Autodesk Fusion 360 part; units mm, degrees
note: some values were not read from the file. Chosen so that the rebuilt part matches the saved one: which face or edge a step refers to; which pieces of a blend or face edit are solid. Set by a fixed rule: which sketch regions a step uses.
(part 2 of 2)
sketch "Sketch14" plane through (0, 6.1, 0) normal (0, 1, 0) x (-1, 0, 0)
  line L0 (1, 7.8) -> (-21.04, 7.8)
  line L1 (-20.84, 4.25) -> (0.8, 4.25) construction
  line L2 (-10.02, 7.8) -> (-10.02, 0.2) construction
  spline S0 degree 3 poles (-10.1584, 7.1337) (-10.2189, 7.0606) (-10.2819, 6.9799) (-10.302, 6.9572) knots 0 0 0 0 1 1 1 1
  spline S1 degree 3 poles (-10.302, 6.9572) (-10.3373, 6.9144) (-10.3222, 6.9119) (-10.0172, 6.9119) knots 0 0 0 0 1 1 1 1
  line L3 (-10.0172, 6.9119) -> (-9.697, 6.9119)
  line L4 (-9.697, 6.9119) -> (-9.818, 7.0581)
  spline S2 degree 3 poles (-9.818, 7.0581) (-9.9441, 7.2068) (-10.0021, 7.2648) (-10.0323, 7.2648) knots 0 0 0 0 1 1 1 1
  spline S3 degree 3 poles (-10.0323, 7.2648) (-10.0424, 7.2648) (-10.0979, 7.2043) (-10.1584, 7.1337) knots 0 0 0 0 1 1 1 1
  spline S4 degree 3 poles (-11.6481, 6.2766) (-12.0111, 5.8405) (-12.0968, 5.7347) (-12.0968, 5.7246) knots 0 0 0 0 1 1 1 1
  spline S5 degree 3 poles (-12.0968, 5.7246) (-12.0968, 5.7195) (-11.9254, 5.7195) (-11.7162, 5.7271) knots 0 0 0 0 1 1 1 1
  line L5 (-11.7162, 5.7271) -> (-11.3381, 5.7397)
  line L6 (-11.3381, 5.7397) -> (-11.3381, 6.0372)
  spline S6 degree 3 poles (-11.3381, 6.0372) (-11.3381, 6.1985) (-11.3381, 6.3825) (-11.3406, 6.4455) knots 0 0 0 0 1 1 1 1
  spline S7 degree 3 poles (-11.3406, 6.4455) (-11.3406, 6.5262) (-11.3507, 6.559) (-11.3759, 6.559) knots 0 0 0 0 1 1 1 1
  spline S8 degree 3 poles (-11.3759, 6.559) (-11.3961, 6.559) (-11.5196, 6.4304) (-11.6481, 6.2766) knots 0 0 0 0 1 1 1 1
  spline S9 degree 3 poles (-10.2567, 6.327) (-10.36, 6.201) (-10.5188, 6.017) (-10.6096, 5.9187) knots 0 0 0 0 1 1 1 1
  line L7 (-10.6096, 5.9187) -> (-10.7734, 5.7397)
  line L8 (-10.7734, 5.7397) -> (-10.3877, 5.7321)
  spline S10 degree 3 poles (-10.3877, 5.7321) (-10.176, 5.7296) (-9.8357, 5.7296) (-9.6315, 5.7321) knots 0 0 0 0 1 1 1 1
  line L9 (-9.6315, 5.7321) -> (-9.261, 5.7397)
  line L10 (-9.261, 5.7397) -> (-9.4248, 5.9187)
  spline S11 degree 3 poles (-9.4248, 5.9187) (-9.5156, 6.0145) (-9.6769, 6.201) (-9.7853, 6.327) knots 0 0 0 0 1 1 1 1
  spline S12 degree 3 poles (-9.7853, 6.327) (-9.8937, 6.4556) (-9.9995, 6.559) (-10.0248, 6.559) knots 0 0 0 0 1 1 1 1
  spline S13 degree 3 poles (-10.0248, 6.559) (-10.0474, 6.559) (-10.1533, 6.4556) (-10.2567, 6.327) knots 0 0 0 0 1 1 1 1
  spline S14 degree 3 poles (-8.6963, 6.2943) (-8.6963, 6.1481) (-8.6988, 5.9641) (-8.6988, 5.8859) knots 0 0 0 0 1 1 1 1
  line L11 (-8.6988, 5.8859) -> (-8.7013, 5.7397)
  line L12 (-8.7013, 5.7397) -> (-8.3182, 5.7271)
  spline S15 degree 3 poles (-8.3182, 5.7271) (-8.109, 5.7195) (-7.9375, 5.7195) (-7.9375, 5.7271) knots 0 0 0 0 1 1 1 1
  spline S16 degree 3 poles (-7.9375, 5.7271) (-7.9401, 5.7649) (-8.6257, 6.559) (-8.656, 6.559) knots 0 0 0 0 1 1 1 1
  spline S17 degree 3 poles (-8.656, 6.559) (-8.6862, 6.559) (-8.6938, 6.5111) (-8.6963, 6.2943) knots 0 0 0 0 1 1 1 1
  spline S18 degree 3 poles (-11.5171, 5.1927) (-11.5902, 5.1045) (-11.6683, 5.0162) (-11.691, 4.9961) knots 0 0 0 0 1 1 1 1
  spline S19 degree 3 poles (-11.691, 4.9961) (-11.7137, 4.9759) (-11.8246, 4.8473) (-11.938, 4.7112) knots 0 0 0 0 1 1 1 1
  spline S20 degree 3 poles (-11.938, 4.7112) (-12.1624, 4.444) (-12.2128, 4.3306) (-12.1876, 4.144) knots 0 0 0 0 1 1 1 1
  spline S21 degree 3 poles (-12.1876, 4.144) (-12.1674, 4.0029) (-12.1397, 3.955) (-12.0288, 3.8693) knots 0 0 0 0 1 1 1 1
  spline S22 degree 3 poles (-12.0288, 3.8693) (-11.9481, 3.8063) (-11.9153, 3.7987) (-11.7591, 3.7987) knots 0 0 0 0 1 1 1 1
  spline S23 degree 3 poles (-11.7591, 3.7987) (-11.6607, 3.7987) (-11.5498, 3.8063) (-11.5095, 3.8189) knots 0 0 0 0 1 1 1 1
  spline S24 degree 3 poles (-11.5095, 3.8189) (-11.4213, 3.8441) (-11.4187, 3.8012) (-11.5045, 3.6348) knots 0 0 0 0 1 1 1 1
  line L13 (-11.5045, 3.6348) -> (-11.5675, 3.5088)
  line L14 (-11.5675, 3.5088) -> (-11.4792, 3.5063)
  spline S25 degree 3 poles (-11.4792, 3.5063) (-11.4314, 3.5038) (-11.3784, 3.5012) (-11.3658, 3.4987) knots 0 0 0 0 1 1 1 1
  spline S26 degree 3 poles (-11.3658, 3.4987) (-11.3482, 3.4962) (-11.3381, 3.8088) (-11.333, 4.4239) knots 0 0 0 0 1 1 1 1
  spline S27 degree 3 poles (-11.333, 4.4239) (-11.3305, 5.0818) (-11.3356, 5.349) (-11.3557, 5.349) knots 0 0 0 0 1 1 1 1
  spline S28 degree 3 poles (-11.3557, 5.349) (-11.3709, 5.349) (-11.444, 5.2784) (-11.5171, 5.1927) knots 0 0 0 0 1 1 1 1
  spline S29 degree 3 poles (-10.413, 4.9557) (-10.597, 4.739) (-10.781, 4.5096) (-10.8188, 4.4465) knots 0 0 0 0 1 1 1 1
  spline S30 degree 3 poles (-10.8188, 4.4465) (-10.96, 4.2247) (-10.8919, 3.9903) (-10.6474, 3.8466) knots 0 0 0 0 1 1 1 1
  spline S31 degree 3 poles (-10.6474, 3.8466) (-10.544, 3.7861) (-10.5138, 3.7811) (-10.3751, 3.7937) knots 0 0 0 0 1 1 1 1
  spline S32 degree 3 poles (-10.3751, 3.7937) (-10.2894, 3.8012) (-10.1911, 3.8163) (-10.1584, 3.8264) knots 0 0 0 0 1 1 1 1
  spline S33 degree 3 poles (-10.1584, 3.8264) (-10.1029, 3.8441) (-10.1004, 3.839) (-10.1155, 3.7735) knots 0 0 0 0 1 1 1 1
  spline S34 degree 3 poles (-10.1155, 3.7735) (-10.1306, 3.713) (-10.1936, 3.5567) (-10.2239, 3.5088) knots 0 0 0 0 1 1 1 1
  spline S35 degree 3 poles (-10.2239, 3.5088) (-10.2289, 3.5012) (-10.1357, 3.4962) (-10.0172, 3.4962) knots 0 0 0 0 1 1 1 1
  spline S36 degree 3 poles (-10.0172, 3.4962) (-9.8987, 3.4962) (-9.8054, 3.5012) (-9.8105, 3.5088) knots 0 0 0 0 1 1 1 1
  spline S37 degree 3 poles (-9.8105, 3.5088) (-9.8483, 3.5743) (-9.929, 3.7735) (-9.929, 3.8037) knots 0 0 0 0 1 1 1 1
  spline S38 degree 3 poles (-9.929, 3.8037) (-9.929, 3.8315) (-9.9138, 3.839) (-9.871, 3.8264) knots 0 0 0 0 1 1 1 1
  spline S39 degree 3 poles (-9.871, 3.8264) (-9.8407, 3.8163) (-9.7424, 3.8012) (-9.6517, 3.7937) knots 0 0 0 0 1 1 1 1
  spline S40 degree 3 poles (-9.6517, 3.7937) (-9.4979, 3.7811) (-9.4803, 3.7861) (-9.3643, 3.8642) knots 0 0 0 0 1 1 1 1
  spline S41 degree 3 poles (-9.3643, 3.8642) (-9.2156, 3.9676) (-9.1475, 4.0861) (-9.1475, 4.2398) knots 0 0 0 0 1 1 1 1
  spline S42 degree 3 poles (-9.1475, 4.2398) (-9.1475, 4.3835) (-9.1904, 4.4491) (-9.6214, 4.9557) knots 0 0 0 0 1 1 1 1
  spline S43 degree 3 poles (-9.6214, 4.9557) (-9.8811, 5.2608) (-9.9693, 5.349) (-10.0172, 5.349) knots 0 0 0 0 1 1 1 1
  spline S44 degree 3 poles (-10.0172, 5.349) (-10.0651, 5.349) (-10.1533, 5.2608) (-10.413, 4.9557) knots 0 0 0 0 1 1 1 1
  line L15 (-8.7064, 4.4289) -> (-8.7064, 3.5088)
  line L16 (-8.7064, 3.5088) -> (-8.5829, 3.5088)
  line L17 (-8.5829, 3.5088) -> (-8.4619, 3.5088)
  line L18 (-8.4619, 3.5088) -> (-8.5047, 3.5743)
  spline S45 degree 3 poles (-8.5047, 3.5743) (-8.5274, 3.6096) (-8.5627, 3.6853) (-8.5829, 3.7407) knots 0 0 0 0 1 1 1 1
  spline S46 degree 3 poles (-8.5829, 3.7407) (-8.6182, 3.8415) (-8.6182, 3.8415) (-8.5602, 3.8239) knots 0 0 0 0 1 1 1 1
  spline S47 degree 3 poles (-8.5602, 3.8239) (-8.5299, 3.8163) (-8.424, 3.8012) (-8.3283, 3.7962) knots 0 0 0 0 1 1 1 1
  spline S48 degree 3 poles (-8.3283, 3.7962) (-8.177, 3.7861) (-8.1392, 3.7911) (-8.0535, 3.8415) knots 0 0 0 0 1 1 1 1
  spline S49 degree 3 poles (-8.0535, 3.8415) (-7.8922, 3.9373) (-7.8493, 4.0155) (-7.8518, 4.2096) knots 0 0 0 0 1 1 1 1
  spline S50 degree 3 poles (-7.8518, 4.2096) (-7.8518, 4.3029) (-7.8644, 4.4037) (-7.8821, 4.4314) knots 0 0 0 0 1 1 1 1
  spline S51 degree 3 poles (-7.8821, 4.4314) (-7.9451, 4.5474) (-8.6434, 5.349) (-8.6812, 5.349) knots 0 0 0 0 1 1 1 1
  spline S52 degree 3 poles (-8.6812, 5.349) (-8.6988, 5.349) (-8.7064, 5.0339) (-8.7064, 4.4289) knots 0 0 0 0 1 1 1 1
  spline S53 degree 3 poles (-12.6917, 4.56) (-12.8077, 4.4289) (-12.8682, 4.26) (-12.8405, 4.144) knots 0 0 0 0 1 1 1 1
  spline S54 degree 3 poles (-12.8405, 4.144) (-12.8329, 4.1012) (-12.7724, 4.013) (-12.7069, 3.9449) knots 0 0 0 0 1 1 1 1
  line L19 (-12.7069, 3.9449) -> (-12.5884, 3.8239)
  line L20 (-12.5884, 3.8239) -> (-12.5808, 4.0457)
  spline S55 degree 3 poles (-12.5808, 4.0457) (-12.5783, 4.1667) (-12.5783, 4.3608) (-12.5808, 4.4717) knots 0 0 0 0 1 1 1 1
  line L21 (-12.5808, 4.4717) -> (-12.5884, 4.6785)
  line L22 (-12.5884, 4.6785) -> (-12.6917, 4.56)
  line L23 (-7.4586, 4.255) -> (-7.4586, 3.834)
  line L24 (-7.4586, 3.834) -> (-7.3855, 3.8844)
  spline S56 degree 3 poles (-7.3855, 3.8844) (-7.1435, 4.0583) (-7.141, 4.376) (-7.3804, 4.6028) knots 0 0 0 0 1 1 1 1
  line L25 (-7.3804, 4.6028) -> (-7.4586, 4.6785)
  line L26 (-7.4586, 4.6785) -> (-7.4586, 4.255)
  spline S57 degree 3 poles (-10.8692, 3.1382) (-10.8793, 3.1307) (-10.8869, 3.0677) (-10.8869, 2.9996) knots 0 0 0 0 1 1 1 1
  spline S58 degree 3 poles (-10.8869, 2.9996) (-10.8869, 2.8559) (-10.8138, 2.7374) (-10.6676, 2.6492) knots 0 0 0 0 1 1 1 1
  spline S59 degree 3 poles (-10.6676, 2.6492) (-10.5869, 2.5988) (-10.5566, 2.5963) (-10.3399, 2.6089) knots 0 0 0 0 1 1 1 1
  spline S60 degree 3 poles (-10.3399, 2.6089) (-10.0701, 2.6265) (-10.0777, 2.6366) (-10.1836, 2.4148) knots 0 0 0 0 1 1 1 1
  spline S61 degree 3 poles (-10.1836, 2.4148) (-10.2113, 2.3593) (-10.2315, 2.3114) (-10.2315, 2.3064) knots 0 0 0 0 1 1 1 1
  spline S62 degree 3 poles (-10.2315, 2.3064) (-10.2315, 2.3013) (-10.1357, 2.2988) (-10.0197, 2.2988) knots 0 0 0 0 1 1 1 1
  line L27 (-10.0197, 2.2988) -> (-9.8054, 2.2988)
  line L28 (-9.8054, 2.2988) -> (-9.8685, 2.4375)
  spline S63 degree 3 poles (-9.8685, 2.4375) (-9.9012, 2.5156) (-9.929, 2.5887) (-9.929, 2.6013) knots 0 0 0 0 1 1 1 1
  spline S64 degree 3 poles (-9.929, 2.6013) (-9.929, 2.6164) (-9.8332, 2.619) (-9.6895, 2.6089) knots 0 0 0 0 1 1 1 1
  spline S65 degree 3 poles (-9.6895, 2.6089) (-9.4626, 2.5938) (-9.4475, 2.5963) (-9.3517, 2.6593) knots 0 0 0 0 1 1 1 1
  spline S66 degree 3 poles (-9.3517, 2.6593) (-9.2105, 2.7551) (-9.1425, 2.8736) (-9.1526, 3.0223) knots 0 0 0 0 1 1 1 1
  line L29 (-9.1526, 3.0223) -> (-9.1601, 3.1433)
  line L30 (-9.1601, 3.1433) -> (-10.0071, 3.1509)
  spline S67 degree 3 poles (-10.0071, 3.1509) (-10.4709, 3.1534) (-10.8591, 3.1483) (-10.8692, 3.1382) knots 0 0 0 0 1 1 1 1
  spline S68 degree 3 poles (-8.6761, 3.1382) (-8.6862, 3.1307) (-8.6938, 2.9366) (-8.6938, 2.7097) knots 0 0 0 0 1 1 1 1
  line L31 (-8.6938, 2.7097) -> (-8.6938, 2.2988)
  line L32 (-8.6938, 2.2988) -> (-8.5703, 2.2988)
  line L33 (-8.5703, 2.2988) -> (-8.4442, 2.2988)
  line L34 (-8.4442, 2.2988) -> (-8.5198, 2.44)
  spline S69 degree 3 poles (-8.5198, 2.44) (-8.6257, 2.6417) (-8.6232, 2.6442) (-8.4215, 2.6164) knots 0 0 0 0 1 1 1 1
  spline S70 degree 3 poles (-8.4215, 2.6164) (-8.1871, 2.5837) (-8.0787, 2.6089) (-7.9552, 2.7248) knots 0 0 0 0 1 1 1 1
  spline S71 degree 3 poles (-7.9552, 2.7248) (-7.8569, 2.8156) (-7.8518, 2.8307) (-7.8417, 2.9895) knots 0 0 0 0 1 1 1 1
  line L35 (-7.8417, 2.9895) -> (-7.8317, 3.1559)
  line L36 (-7.8317, 3.1559) -> (-8.2451, 3.1559)
  spline S72 degree 3 poles (-8.2451, 3.1559) (-8.4745, 3.1559) (-8.6686, 3.1483) (-8.6761, 3.1382) knots 0 0 0 0 1 1 1 1
  spline S73 degree 3 poles (-12.1977, 3.0097) (-12.1977, 2.8736) (-12.1347, 2.7576) (-12.0137, 2.6669) knots 0 0 0 0 1 1 1 1
  spline S74 degree 3 poles (-12.0137, 2.6669) (-11.9506, 2.6215) (-11.9078, 2.6139) (-11.696, 2.6164) knots 0 0 0 0 1 1 1 1
  line L37 (-11.696, 2.6164) -> (-11.449, 2.619)
  line L38 (-11.449, 2.619) -> (-11.4515, 2.5534)
  spline S75 degree 3 poles (-11.4515, 2.5534) (-11.4515, 2.5181) (-11.4616, 2.4828) (-11.4692, 2.4753) knots 0 0 0 0 1 1 1 1
  spline S76 degree 3 poles (-11.4692, 2.4753) (-11.4792, 2.4677) (-11.5095, 2.4223) (-11.5372, 2.3719) knots 0 0 0 0 1 1 1 1
  line L39 (-11.5372, 2.3719) -> (-11.5876, 2.2812)
  line L40 (-11.5876, 2.2812) -> (-11.4717, 2.2938)
  spline S77 degree 3 poles (-11.4717, 2.2938) (-11.4061, 2.2988) (-11.3507, 2.3064) (-11.3482, 2.3089) knots 0 0 0 0 1 1 1 1
  spline S78 degree 3 poles (-11.3482, 2.3089) (-11.3456, 2.3114) (-11.3406, 2.4954) (-11.3381, 2.7148) knots 0 0 0 0 1 1 1 1
  line L41 (-11.3381, 2.7148) -> (-11.3356, 3.1181)
  line L42 (-11.3356, 3.1181) -> (-11.7666, 3.1256)
  line L43 (-11.7666, 3.1256) -> (-12.1977, 3.1307)
  line L44 (-12.1977, 3.1307) -> (-12.1977, 3.0097)
  spline S79 degree 3 poles (-10.1054, 1.9257) (-10.1054, 1.9005) (-10.1382, 1.8174) (-10.181, 1.7367) knots 0 0 0 0 1 1 1 1
  line L45 (-10.181, 1.7367) -> (-10.2541, 1.593)
  line L46 (-10.2541, 1.593) -> (-10.0298, 1.593)
  spline S80 degree 3 poles (-10.0298, 1.593) (-9.9038, 1.593) (-9.8029, 1.598) (-9.8029, 1.6031) knots 0 0 0 0 1 1 1 1
  spline S81 degree 3 poles (-9.8029, 1.6031) (-9.8029, 1.6081) (-9.8307, 1.6737) (-9.8659, 1.7493) knots 0 0 0 0 1 1 1 1
  spline S82 degree 3 poles (-9.8659, 1.7493) (-9.9012, 1.8224) (-9.929, 1.9031) (-9.929, 1.9283) knots 0 0 0 0 1 1 1 1
  spline S83 degree 3 poles (-9.929, 1.9283) (-9.929, 1.961) (-9.9491, 1.9711) (-10.0172, 1.9711) knots 0 0 0 0 1 1 1 1
  spline S84 degree 3 poles (-10.0172, 1.9711) (-10.0853, 1.9711) (-10.1054, 1.961) (-10.1054, 1.9257) knots 0 0 0 0 1 1 1 1
  line L47 (-21.04, 7.8) -> (-21.04, 0)
  line L48 (-21.04, 0) -> (1, 0)
  line L49 (1, 0) -> (1, 7.8)
  constraint midpoint L0 L2.start
extrude "Extrude23" add sketch "Sketch14" along normal blind 0.3 contours S0 S1 L3 L4 S2 S3 | S4 S5 L5 L6 S6 S7 S8 | S9 L7 L8 S10 L9 L10 S11 S12 S13 | S14 L11 L12 S15 S16 S17 | S18 S19 S20 S21 S22 S23 S24 L13 L14 S25 S26 S27 S28 | S29 S30 S31 S32 S33 S34 S35 S36 S37 S38 S39 S40 S41 S42 S43 S44 | L15 L16 L17 L18 S45 S46 S47 S48 S49 S50 S51 S52 | S53 S54 L19 L20 S55 L21 L22 | L23 L24 S56 L25 L26 | S57 S58 S59 S60 S61 S62 L27 L28 S63 S64 S65 S66 L29 L30 S67 | S68 L31 L32 L33 L34 S69 S70 S71 L35 L36 S72 | S73 S74 L37 L38 S75 S76 L39 L40 S77 S78 L41 L42 L43 L44 | S79 L45 L46 S80 S81 S82 S83 S84
extrude "Extrude24" cut 1 faces at (-0.8348, -0.8228, 0.2) along direction (0, 0, -1) blind 3
sketch "Sketch15" plane through (21.04, 0, 0) normal (1, 0, 0) x (0, 1, 0)
  line L0 (6.1, 7.8) -> (-1, 7.8)
  line L1 (2.4054, 2.652) -> (3.5519, 5.6541)
  line L2 (3.5519, 5.6541) -> (3.9796, 5.6549)
  line L3 (3.9796, 5.6549) -> (5.2131, 2.6572)
  line L4 (5.2131, 2.6572) -> (4.7608, 2.6564)
  line L5 (4.7608, 2.6564) -> (4.4092, 3.5643)
  line L6 (4.4092, 3.5643) -> (3.1547, 3.562)
  line L7 (3.1547, 3.562) -> (2.827, 2.6528)
  line L8 (2.827, 2.6528) -> (2.4054, 2.652)
  line L9 (-0.1973, 3.611) -> (0.1771, 3.6444)
  spline S0 degree 3 poles (0.1771, 3.6444) (0.1878, 3.5746) (0.2078, 3.444) (0.2711, 3.3282) (0.3006, 3.2742) knots 0 0 0 0 0.020982 0.039288 0.039288 0.039288 0.039288
  spline S1 degree 3 poles (0.3006, 3.2742) (0.3399, 3.2279) (0.424, 3.1287) (0.5413, 3.0718) (0.6039, 3.0415) knots 0 0 0 0 0.018019 0.038604 0.038604 0.038604 0.038604
  spline S2 degree 3 poles (0.6039, 3.0415) (0.6757, 3.016) (0.8246, 2.9631) (0.9826, 2.9573) (1.0645, 2.9544) knots 0 0 0 0 0.022722 0.047123 0.047123 0.047123 0.047123
  spline S3 degree 3 poles (1.0645, 2.9544) (1.1363, 2.9567) (1.2732, 2.9612) (1.4035, 3.0029) (1.4654, 3.0227) knots 0 0 0 0 0.021451 0.040849 0.040849 0.040849 0.040849
  spline S4 degree 3 poles (1.4654, 3.0227) (1.5185, 3.0458) (1.6177, 3.0891) (1.6895, 3.1698) (1.7229, 3.2073) knots 0 0 0 0 0.017118 0.032023 0.032023 0.032023 0.032023
  spline S5 degree 3 poles (1.7229, 3.2073) (1.7479, 3.2474) (1.7972, 3.3266) (1.8047, 3.4195) (1.8084, 3.4653) knots 0 0 0 0 0.013958 0.027533 0.027533 0.027533 0.027533
  spline S6 degree 3 poles (1.8084, 3.4653) (1.8051, 3.5105) (1.7987, 3.5995) (1.75, 3.6741) (1.7261, 3.7107) knots 0 0 0 0 0.013357 0.026267 0.026267 0.026267 0.026267
  spline S7 degree 3 poles (1.7261, 3.7107) (1.6915, 3.7457) (1.6142, 3.8238) (1.5121, 3.8653) (1.4556, 3.8883) knots 0 0 0 0 0.014598 0.03265 0.03265 0.03265 0.03265
  spline S8 degree 3 poles (1.4556, 3.8883) (1.3911, 3.9087) (1.2152, 3.9646) (1.0352, 4.0062) (0.9212, 4.0326) knots 0 0 0 0 0.020292 0.05537 0.05537 0.05537 0.05537
  spline S9 degree 3 poles (0.9212, 4.0326) (0.8028, 4.0609) (0.6046, 4.1084) (0.4171, 4.1878) (0.3418, 4.2197) knots 0 0 0 0 0.036466 0.060986 0.060986 0.060986 0.060986
  spline S10 degree 3 poles (0.3418, 4.2197) (0.2757, 4.2577) (0.1504, 4.3297) (0.0618, 4.4436) (0.02, 4.4974) knots 0 0 0 0 0.022603 0.04287 0.04287 0.04287 0.04287
  spline S11 degree 3 poles (0.02, 4.4974) (-0.0106, 4.5553) (-0.0724, 4.6725) (-0.0808, 4.8048) (-0.0851, 4.8717) knots 0 0 0 0 0.019401 0.03927 0.03927 0.03927 0.03927
  spline S12 degree 3 poles (-0.0851, 4.8717) (-0.0797, 4.9465) (-0.0687, 5.0973) (0.0056, 5.2291) (0.043, 5.2956) knots 0 0 0 0 0.022183 0.04477 0.04477 0.04477 0.04477
  spline S13 degree 3 poles (0.043, 5.2956) (0.0921, 5.3584) (0.1937, 5.4882) (0.3423, 5.56) (0.419, 5.5971) knots 0 0 0 0 0.023577 0.048769 0.048769 0.048769 0.048769
  spline S14 degree 3 poles (0.419, 5.5971) (0.5053, 5.6271) (0.6835, 5.689) (0.872, 5.6966) (0.9693, 5.7005) knots 0 0 0 0 0.027246 0.056264 0.056264 0.056264 0.056264
  spline S15 degree 3 poles (0.9693, 5.7005) (1.0749, 5.6971) (1.2762, 5.6906) (1.4664, 5.6245) (1.5568, 5.5931) knots 0 0 0 0 0.031478 0.060031 0.060031 0.060031 0.060031
  spline S16 degree 3 poles (1.5568, 5.5931) (1.6365, 5.5545) (1.7917, 5.4795) (1.8984, 5.3444) (1.9503, 5.2787) knots 0 0 0 0 0.026183 0.050954 0.050954 0.050954 0.050954
  spline S17 degree 3 poles (1.9503, 5.2787) (1.9909, 5.2062) (2.0732, 5.0592) (2.09, 4.8914) (2.0985, 4.8062) knots 0 0 0 0 0.024624 0.04999 0.04999 0.04999 0.04999
  line L10 (2.0985, 4.8062) -> (1.7179, 4.7769)
  spline S18 degree 3 poles (1.7179, 4.7769) (1.7034, 4.8642) (1.676, 5.0286) (1.562, 5.1495) (1.5084, 5.2062) knots 0 0 0 0 0.025863 0.048747 0.048747 0.048747 0.048747
  spline S19 degree 3 poles (1.5084, 5.2062) (1.4373, 5.2483) (1.2771, 5.3432) (1.0902, 5.3479) (0.9863, 5.3506) knots 0 0 0 0 0.024412 0.054967 0.054967 0.054967 0.054967
  spline S20 degree 3 poles (0.9863, 5.3506) (0.8799, 5.3487) (0.6931, 5.3454) (0.5305, 5.2553) (0.4606, 5.2166) knots 0 0 0 0 0.031333 0.054977 0.054977 0.054977 0.054977
  spline S21 degree 3 poles (0.4606, 5.2166) (0.413, 5.1716) (0.3209, 5.0848) (0.3051, 4.9595) (0.2975, 4.8991) knots 0 0 0 0 0.018984 0.036703 0.036703 0.036703 0.036703
  spline S22 degree 3 poles (0.2975, 4.8991) (0.3023, 4.8477) (0.3118, 4.746) (0.3806, 4.6706) (0.4147, 4.6332) knots 0 0 0 0 0.01502 0.029764 0.029764 0.029764 0.029764
  spline S23 degree 3 poles (0.4147, 4.6332) (0.4826, 4.5954) (0.6692, 4.4916) (0.8791, 4.4475) (1.0126, 4.4195) knots 0 0 0 0 0.023224 0.0638 0.0638 0.0638 0.0638
  spline S24 degree 3 poles (1.0126, 4.4195) (1.15, 4.3894) (1.3758, 4.34) (1.593, 4.2613) (1.678, 4.2304) knots 0 0 0 0 0.042125 0.069241 0.069241 0.069241 0.069241
  spline S25 degree 3 poles (1.678, 4.2304) (1.7581, 4.1899) (1.9082, 4.114) (2.0154, 3.9846) (2.0654, 3.9242) knots 0 0 0 0 0.026576 0.049849 0.049849 0.049849 0.049849
  spline S26 degree 3 poles (2.0654, 3.9242) (2.1019, 3.8596) (2.1766, 3.7276) (2.1861, 3.5762) (2.191, 3.4988) knots 0 0 0 0 0.021947 0.044875 0.044875 0.044875 0.044875
  spline S27 degree 3 poles (2.191, 3.4988) (2.1851, 3.4196) (2.1731, 3.2587) (2.0946, 3.1178) (2.0547, 3.0463) knots 0 0 0 0 0.023529 0.047766 0.047766 0.047766 0.047766
  spline S28 degree 3 poles (2.0547, 3.0463) (2.0028, 2.9792) (1.8956, 2.8405) (1.7405, 2.7584) (1.6604, 2.7161) knots 0 0 0 0 0.025147 0.051964 0.051964 0.051964 0.051964
  spline S29 degree 3 poles (1.6604, 2.7161) (1.5708, 2.6819) (1.385, 2.6111) (1.1863, 2.6027) (1.0836, 2.5983) knots 0 0 0 0 0.028588 0.059219 0.059219 0.059219 0.059219
  spline S30 degree 3 poles (1.0836, 2.5983) (0.9575, 2.6013) (0.7236, 2.6069) (0.502, 2.6814) (0.3998, 2.7158) knots 0 0 0 0 0.037566 0.069723 0.069723 0.069723 0.069723
  spline S31 degree 3 poles (0.3998, 2.7158) (0.3136, 2.7596) (0.1431, 2.8462) (0.0255, 2.9967) (-0.0326, 3.071) knots 0 0 0 0 0.028647 0.056577 0.056577 0.056577 0.056577
  spline S32 degree 3 poles (-0.0326, 3.071) (-0.0785, 3.154) (-0.1715, 3.3222) (-0.1887, 3.5138) (-0.1973, 3.611) knots 0 0 0 0 0.028107 0.057006 0.057006 0.057006 0.057006
  circle A0 centre (0.9212, 3.8883) radius 4.8997
  line L11 (-1, 7.8) -> (-1, 0)
  line L12 (-1, 0) -> (6.1, 0)
  line L13 (6.1, 0) -> (6.1, 7.8)
extrude "Extrude25" cut 1 faces at (6.5133, 5.9333, 0) along direction (0, 0, 1) blind 0.5
fillet "Fillet8" radius 0.2 17 edges at (21.04, 6.1, 4.15) (20.9814, 6.0414, 7.9414) (10.02, 6.1, 0.5) (-1, 6.1, 4.15) (-0.9414, 6.0414, 7.9414) (-1, 2.8158, 0.5) (-1, -0.4685, 4.15) (-0.9414, -0.4454, 7.9414) (-0.479, -0.9414, 7.9414) (-0.5045, -1, 4.15) (-0.7523, -0.7342, 0.5) (3.8032, -1, 0.5) (17.7364, -1, 0.5) (11.1394, -1, 0.5) (21.04, -1, 4.15) (20.9814, -0.9414, 7.9414) (21.04, 2.55, 0.5)
equation "LEDWidth = 5.1 mm"
equation "LEDHeight = 7 mm"
equation "LEDLength = 2.1 mm"
equation "d8 = LEDLength"
equation "d9 = LEDWidth"
equation "Pitch = 2.54 mm" comment "Standard Breadboard Pitch"
equation "d30 = Pitch"
equation "d33 = LEDLength"
equation "d34 = LEDWidth"
equation "d38 = Pitch"
equation "d50 = LEDHeight + 0.5 mm"
equation "d57 = Pitch"
equation "d58 = Pitch"
equation "d59 = Pitch"
equation "d60 = Pitch"
equation "d61 = Pitch"
equation "d62 = Pitch"
equation "d63 = Pitch"
equation "d64 = LEDLength - 0.5 mm"
equation "d65 = LEDWidth - 0.5 mm"
equation "d66 = LEDLength - 0.5 mm"
equation "d67 = LEDWidth - 0.5 mm"
equation "d68 = LEDLength - 0.5 mm"
equation "d69 = LEDWidth - 0.5 mm"
equation "d70 = LEDLength - 0.5 mm"
equation "d71 = LEDWidth - 0.5 mm"
equation "d72 = LEDLength - 0.5 mm"
equation "d73 = LEDWidth - 0.5 mm"
equation "d74 = LEDLength - 0.5 mm"
equation "d75 = LEDWidth - 0.5 mm"
equation "d76 = LEDLength - 0.5 mm"
equation "d77 = LEDWidth - 0.5 mm"
equation "d78 = LEDLength - 0.5 mm"
equation "d79 = LEDWidth - 0.5 mm"
equation "TextExr = 0.3 mm"
equation "d113 = TextExr"
equation "d117 = TextExr"
equation "d135 = -LEDHeight - 1 mm"
equation "d153 = TextExr"
equation "d155 = TextExr"
